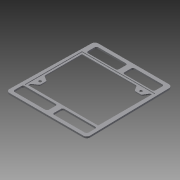
# Autodesk Inventor part: control pod layer b
Saved by Autodesk Inventor 2014 SP1 (Build 180222100, 222)
## iProperties
Created: 2017-06-28
Part Number: control pod layer b
Material: Generic
Document SubType Name: Modeling
Designer: kteo17
Density: 1 g/cm^3
Appearance: Default
Author: kteo17
Autodesk Inventor part; units mm, degrees
ref_plane "YZ Plane" through (0, 0, 0) normal (1, 0, 0) x (0, 1, 0)
ref_plane "XZ Plane" through (0, 0, 0) normal (0, 1, 0) x (-1, 0, 0)
ref_plane "XY Plane" through (0, 0, 0) normal (0, 0, 1) x (1, 0, 0)
sketch "Sketch1" plane through (0, 0, 0) normal (0, 0, 1) x (1, 0, 0)
  line L0 (3.175, 0) -> (146.685, 0)
  line L1 (149.86, 161.925) -> (0, 161.925)
  line L2 (0, 161.925) -> (3.175, 0)
  line L3 (149.86, 161.925) -> (146.685, 0)
  point P0 (0, 0)
  dimension "d74" = 161.925
  dimension "d75" = 143.51
  dimension "d76" = 149.86
  constraints: 8 end point, 1 horizontal, 1 parallel
  measures "d74" distance between parallel lines of L0 L1
  measures "d75" distance of L0.start L0.end
  measures "d76" distance of L1.start L1.end
extrude "Extrusion1" add sketch "Sketch1" along normal blind 3.048
fillet "Fillet1" radius 6.35 3 edges at (149.86, 161.925, 1.524) (146.685, 0, 1.524) (0, 161.925, 1.524)
fillet "Fillet4" radius 6.35 1 edges at (3.175, 0, 1.524)
sketch "Sketch21" plane through (0, 0, 3.048) normal (0, 0, 1) x (1, 0, 0)
  arc A0 (149.733, 155.4505) -> (143.3843, 161.925) centre (143.3843, 155.575) ccw projected
  line L0 (143.3843, 139.7) -> (143.3843, 152.4)
  line L1 (6.4757, 152.4) -> (6.4757, 139.7)
  line L2 (79.8843, 152.4) -> (79.8843, 139.7)
  line L3 (69.9757, 152.4) -> (69.9757, 139.7)
  line L4 (140.2093, 155.575) -> (83.0593, 155.575)
  line L5 (66.8007, 155.575) -> (9.6507, 155.575)
  line L6 (9.6507, 136.525) -> (66.8007, 136.525)
  line L7 (83.0593, 136.525) -> (140.2093, 136.525)
  arc A1 (9.6507, 155.575) -> (6.4757, 152.4) centre (9.6507, 152.4) ccw
  arc A2 (6.4757, 139.7) -> (9.6507, 136.525) centre (9.6507, 139.7) ccw
  arc A3 (66.8007, 136.525) -> (69.9757, 139.7) centre (66.8007, 139.7) ccw
  arc A4 (69.9757, 152.4) -> (66.8007, 155.575) centre (66.8007, 152.4) ccw
  arc A5 (83.0593, 155.575) -> (79.8843, 152.4) centre (83.0593, 152.4) ccw
  arc A6 (79.8843, 139.7) -> (83.0593, 136.525) centre (83.0593, 139.7) ccw
  arc A7 (140.2093, 136.525) -> (143.3843, 139.7) centre (140.2093, 139.7) ccw
  arc A8 (143.3843, 152.4) -> (140.2093, 155.575) centre (140.2093, 152.4) ccw
  line L8 (137.6362, 22.225) -> (137.6362, 9.525)
  line L9 (12.2237, 9.525) -> (12.2237, 22.225)
  line L10 (12.2237, 25.4) -> (137.6362, 6.35) construction
  line L11 (137.6362, 25.4) -> (12.2237, 6.35) construction
  line L12 (69.9757, 9.525) -> (69.9757, 22.225)
  line L13 (79.8843, 22.225) -> (79.8843, 9.525)
  line L14 (79.8843, 6.35) -> (69.9757, 25.4) construction
  line L15 (69.9757, 6.35) -> (79.8843, 25.4) construction
  line L16 (15.3987, 25.4) -> (66.8007, 25.4)
  line L17 (83.0593, 25.4) -> (134.4612, 25.4)
  line L18 (134.4612, 6.35) -> (83.0593, 6.35)
  line L19 (66.8007, 6.35) -> (15.3987, 6.35)
  arc A9 (15.3987, 25.4) -> (12.2237, 22.225) centre (15.3987, 22.225) ccw
  arc A10 (12.2237, 9.525) -> (15.3987, 6.35) centre (15.3987, 9.525) ccw
  arc A11 (66.8007, 6.35) -> (69.9757, 9.525) centre (66.8007, 9.525) ccw
  arc A12 (69.9757, 22.225) -> (66.8007, 25.4) centre (66.8007, 22.225) ccw
  arc A13 (83.0593, 25.4) -> (79.8843, 22.225) centre (83.0593, 22.225) ccw
  arc A14 (137.6362, 22.225) -> (134.4612, 25.4) centre (134.4612, 22.225) ccw
  arc A15 (134.4612, 6.35) -> (137.6362, 9.525) centre (134.4612, 9.525) ccw
  arc A16 (79.8843, 9.525) -> (83.0593, 6.35) centre (83.0593, 9.525) ccw
  point P0 (0, 0)
  point P1 (74.93, 15.875)
  dimension "d97" = 3.175
  dimension "d111" = 19.05
  dimension "d112" = 19.05
  dimension "d113" = 63.5
  dimension "d114" = 63.5
  dimension "d131" = 9.9085
  dimension "d141" = 19.05
  dimension "d142" = 3.175
  constraints: 40 end point, 32 point on circle, 32 tangent, 18 point on line, 16 centre point, 14 equal radius, 11 parallel, 8 perpendicular, 4 horizontal, 4 midpoint
  measures "d97" radius of A1
  measures "d111" distance between parallel lines of L6 L5
  measures "d112" distance between parallel lines of L4 L7
  measures "d113" distance between parallel lines of L3 L1
  measures "d114" distance between parallel lines of L0 L2
  measures "d131" distance between parallel lines of L2 L3
  measures "d141" distance of L11.start L10.end
  measures "d142" radius of A9
extrude "Extrusion20" cut sketch "Sketch21" against normal blind 3.048
sketch "Sketch23" plane through (0, 0, 3.048) normal (0, 0, 1) x (1, 0, 0)
  line L0 (142.875, 27.752) -> (6.985, 27.752)
  line L1 (6.985, 27.752) -> (6.985, 133.924)
  line L2 (6.985, 133.924) -> (142.875, 133.924)
  line L3 (142.875, 133.924) -> (142.875, 27.752)
  line L4 (142.875, 27.752) -> (6.985, 133.924) construction
  line L5 (6.985, 27.752) -> (142.875, 133.924) construction
  line L6 (10.16, 130.749) -> (139.7, 130.749)
  line L7 (10.16, 30.927) -> (10.16, 130.749)
  line L8 (139.7, 30.927) -> (10.16, 30.927)
  line L9 (139.7, 130.749) -> (139.7, 30.927)
  point P0 (0, 0)
  point P1 (74.93, 80.838)
  dimension "d129" = 135.89
  dimension "d130" = 106.172
  dimension "d132" = 3.175
  dimension "d133" = 3.175
  dimension "d134" = 3.175
  dimension "d135" = 3.175
  constraints: 20 end point, 6 parallel, 2 midpoint, 1 horizontal, 1 perpendicular
  measures "d129" distance of L1.end L2.end
  measures "d130" distance of L0.end L1.end
  measures "d132" distance between parallel lines of L6 L2
  measures "d133" distance between parallel lines of L1 L7
  measures "d134" distance between parallel lines of L0 L8
  measures "d135" distance between parallel lines of L3 L9
extrude "Extrusion22" cut sketch "Sketch23" against normal blind 3.048 contours L6 L9 L8 L7
sketch "Sketch25" plane through (0, 0, 3.048) normal (0, 0, 1) x (1, 0, 0)
  line L0 (10.16, 30.927) -> (10.16, 130.749) projected
  line L1 (10.16, 130.749) -> (139.7, 130.749) projected
  line L2 (139.7, 130.749) -> (139.7, 30.927) projected
  line L3 (139.7, 30.927) -> (10.16, 30.927) projected
  line L4 (142.875, 133.924) -> (6.985, 133.924)
  line L5 (6.985, 133.924) -> (6.985, 27.752)
  line L6 (6.985, 27.752) -> (142.875, 27.752)
  line L7 (142.875, 27.752) -> (142.875, 133.924)
  point P0 (0, 0)
  dimension "d138" = 3.175
  constraints: 8 end point, 3 other
  measures "d138" distance between parallel lines of L5 L0
extrude "Extrusion23" cut sketch "Sketch25" against normal blind 1.27
sketch "Sketch34" plane through (0, 0, 0) normal (0, 0, -1) x (-1, 0, 0)
  line L0 (-10.16, 130.749) -> (-10.16, 30.927) projected
  line L1 (-10.16, 30.927) -> (-139.7, 30.927) projected
  line L2 (-139.7, 30.927) -> (-139.7, 130.749) projected
  line L3 (-139.7, 130.749) -> (-10.16, 130.749) projected
  line L4 (-6.985, 133.924) -> (-6.985, 27.752)
  line L5 (-6.985, 27.752) -> (-142.875, 27.752)
  line L6 (-142.875, 27.752) -> (-142.875, 133.924)
  line L7 (-142.875, 133.924) -> (-6.985, 133.924)
  circle A0 centre (-134.9375, 113.35) radius 2.413
  line L8 (-129.3495, 117.923) -> (-129.3495, 108.777)
  line L9 (-130.8642, 120.6293) -> (-138.1853, 125.1208)
  line L10 (-130.8642, 106.0708) -> (-138.1853, 101.5793)
  line L11 (-139.7, 127.827) -> (-139.7, 130.749)
  line L12 (-139.7, 98.873) -> (-139.7, 93.6625)
  arc A1 (-139.7, 127.827) -> (-138.1853, 125.1208) centre (-136.525, 127.827) ccw
  arc A2 (-129.3495, 117.923) -> (-130.8642, 120.6293) centre (-132.5245, 117.923) ccw
  arc A3 (-130.8642, 106.0708) -> (-129.3495, 108.777) centre (-132.5245, 108.777) ccw
  arc A4 (-138.1853, 101.5793) -> (-139.7, 98.873) centre (-136.525, 98.873) ccw
  line L13 (-139.7, 127.827) -> (-139.7, 98.873)
  circle A5 centre (-25.654, 35.6895) radius 2.413
  line L14 (-21.081, 41.275) -> (-30.227, 41.275)
  line L15 (-32.9333, 39.7603) -> (-37.4232, 32.4417)
  line L16 (-18.3747, 39.7603) -> (-13.8848, 32.4417)
  line L17 (-40.1295, 30.927) -> (-42.8625, 30.927)
  line L18 (-11.1785, 30.927) -> (-10.16, 30.927)
  arc A6 (-40.1295, 30.927) -> (-37.4232, 32.4417) centre (-40.1295, 34.102) ccw
  arc A7 (-13.8848, 32.4417) -> (-11.1785, 30.927) centre (-11.1785, 34.102) ccw
  arc A8 (-18.3747, 39.7603) -> (-21.081, 41.275) centre (-21.081, 38.1) ccw
  arc A9 (-30.227, 41.275) -> (-32.9333, 39.7603) centre (-30.227, 38.1) ccw
  line L19 (-40.1295, 30.927) -> (-11.1785, 30.927)
  point P0 (0, 0)
  point P1 (-129.3495, 119.7)
  point P2 (-129.3495, 107)
  point P3 (-139.7, 126.05)
  point P4 (-139.7, 100.65)
  point P5 (-19.304, 41.275)
  point P6 (-32.004, 41.275)
  point P7 (-38.3525, 30.927)
  point P8 (-12.9555, 30.927)
  dimension "d223" = 3.175
  dimension "d226" = 4.826
  dimension "d227" = 20.574
  dimension "d228" = 7.9375
  dimension "d231" = 12.7
  dimension "d235" = 3.175
  dimension "d240" = 4.826
  dimension "d241" = 18.669
  dimension "d242" = 7.9375
  dimension "d244" = 12.7
  dimension "d247" = 3.175
  dimension "d248" = 8.127
  dimension "d249" = 8.127
  dimension "d250" = 4.573
  dimension "d251" = 4.573
  dimension "d253" = 5.588
  dimension "d254" = 4.573
  dimension "d255" = 4.573
  constraints: 32 end point, 22 point on line, 20 tangent, 16 point on circle, 10 centre point, 6 equal radius, 4 collinear, 2 perpendicular, 3 other
  measures "d223" distance between parallel lines of L2 L6
  measures "d226" diameter of A0
  measures "d227" distance from line of A0.centre L7
  measures "d228" distance from line of L6 A0.centre
  measures "d231" distance of point (-129.349, 119.7) point (-129.349, 107)
  measures "d235" radius of A1
  measures "d240" diameter of A5
  measures "d241" distance from line of L4 A5.centre
  measures "d242" distance from line of L5 A5.centre
  measures "d244" distance of point (-19.304, 41.275) point (-32.004, 41.275)
  measures "d247" radius of A6
  measures "d248" vertical distance of point (-129.349, 119.7) A1.centre
  measures "d249" vertical distance of point (-129.349, 107) A4.centre
  measures "d250" vertical distance of A3.centre A0.centre
  measures "d251" vertical distance of A0.centre A2.centre
  measures "d253" distance from line of A0.centre L8
  measures "d254" horizontal distance of A5.centre A9.centre
  measures "d255" horizontal distance of A8.centre A5.centre
extrude "Extrusion29" add sketch "Sketch34" against normal blind 1.778 contours L1 A6 L15 A9 L14 A8 L16 A7 | A1 L9 A2 L8 A3 L10 A4 L2
body "Solid1"
